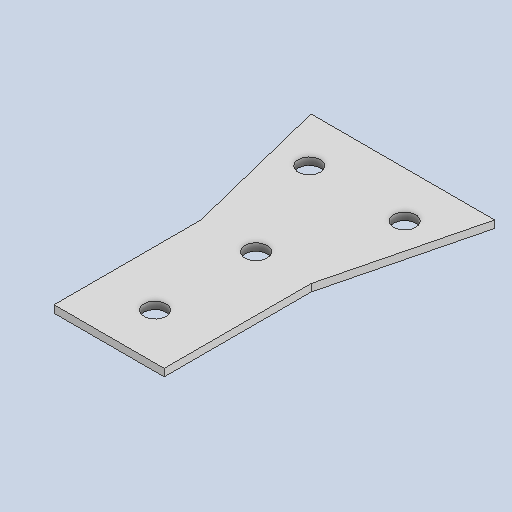
# Autodesk Inventor part: ConnectTx3030_m6
Saved by Autodesk Inventor 2024 (Build 280153000, 153)
## iProperties
Created: 2025-12-08
Part Number: ConnectTx3030_m6
Material: Generic
Document SubType Name: Modeling
Designer: schar
Density: 1 g/cm^3
Appearance: Default
Author: schar
Autodesk Inventor part; units mm, degrees
ref_plane "YZ Plane" through (0, 0, 0) normal (1, 0, 0) x (0, 1, 0)
ref_plane "XZ Plane" through (0, 0, 0) normal (0, 1, 0) x (-1, 0, 0)
ref_plane "XY Plane" through (0, 0, 0) normal (0, 0, 1) x (1, 0, 0)
sketch "Sketch1" plane through (0, 0, 0) normal (0, 1, 0) x (-1, 0, 0)
  line L0 (15, 40) -> (-15, 40)
  line L1 (-15, 40) -> (-15, -40)
  line L2 (-15, -40) -> (15, -40)
  line L3 (15, -40) -> (15, 40)
  line L4 (15, 40) -> (-15, -40) construction
  line L5 (-15, 40) -> (15, -40) construction
  circle A0 centre (0, 0) radius 3
  line L6 (0, 0) -> (0, -27.5)
  line L7 (0, 0) -> (0, 27.5)
  circle A1 centre (0, 27.5) radius 3
  line L8 (-15, -40) -> (-25, -40)
  line L9 (-25, -40) -> (-15, 0)
  line L10 (15, -40) -> (25, -40)
  line L11 (25, -40) -> (15, 0)
  line L12 (0, -27.5) -> (13, -27.5)
  line L13 (0, -27.5) -> (-13, -27.5)
  circle A2 centre (13, -27.5) radius 3
  circle A3 centre (-13, -27.5) radius 3
  dimension "d0" = 30
  dimension "d1" = 80
  dimension "d2" = 6
  dimension "d3" = 27.5
  dimension "d4" = 27.5
  dimension "d5" = 6
  dimension "d6" = 10
  dimension "d7" = 10
  dimension "d8" = 13
  dimension "d9" = 13
  dimension "d10" = 6
  dimension "d11" = 6
  constraints: 28 end point, 4 centre point, 4 coincident, 4 midpoint, 3 horizontal, 3 parallel, 2 vertical, 1 perpendicular, 1 point on line
  measures "d0" distance of L2.end L1.end
  measures "d1" distance of L1.end L0.end
  measures "d2" diameter of A0
  measures "d3" distance of L6.start L6.end
  measures "d4" distance of L6.start L7.end
  measures "d5" diameter of A1
  measures "d6" distance of L1.end L8.end
  measures "d7" distance of L2.end L10.end
  measures "d8" distance of L6.end L12.end
  measures "d9" distance of L6.end L13.end
  measures "d10" diameter of A2
  measures "d11" diameter of A3
extrude "Extrusion1" add sketch "Sketch1" along normal blind 2 contours L3 A2 L12 L13 A3 L1 L0 | L11 L10 L3 A2 | L1 A3 L8 L9 | L3 L2 L1 A3 L13 L12 A2
body "Solid1"
